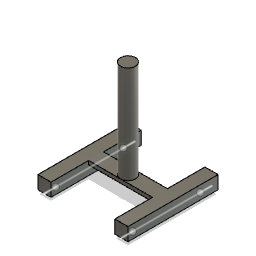
Pedestal (Autodesk Fusion 360 design; units mm, degrees)
Autodesk Fusion 360 part; units mm, degrees
sketch "Sketch1" plane through (0, 0, 0) normal (0, 1, 0) x (1, 0, 0)
  line L0 (609.6, 0) -> (609.6, 609.6)
  line L1 (0, 609.6) -> (0, 0)
  line L2 (0, 0) -> (88.9, 0)
  line L3 (88.9, 609.6) -> (0, 609.6)
  line L4 (0, 609.6) -> (0, 0)
  line L5 (609.6, 609.6) -> (520.7, 609.6)
  line L6 (520.7, -460.804) -> (609.6, -460.804)
  line L7 (609.6, -460.804) -> (609.6, 609.6)
  line L8 (609.6, 304.8) -> (609.6, 355.6)
  line L9 (520.7, 355.6) -> (88.9, 355.6)
  line L10 (0, 355.6) -> (0, 304.8)
  line L11 (609.6, 304.8) -> (609.6, 254)
  line L12 (520.7, 254) -> (88.9, 254)
  line L13 (0, 254) -> (0, 304.8)
  line L14 (88.9, 0) -> (88.9, 254)
  line L15 (88.9, 355.6) -> (88.9, 609.6)
  line L16 (520.7, 609.6) -> (520.7, 355.6)
  line L17 (520.7, 254) -> (520.7, 0)
  line L18 (0, 0) -> (88.9, 0)
  line L19 (520.7, 0) -> (609.6, 0)
  line L20 (609.6, 609.6) -> (520.7, 609.6)
  line L21 (88.9, 609.6) -> (0, 609.6)
  dimension "d1" = 609.6
  dimension "d2" = 609.6
  dimension "d3" = 88.9
  dimension "d4" = 88.9
  dimension "d5" = 50.8
  dimension "d6" = 50.8
  constraint horizontal L18
  constraint vertical L0
  constraint horizontal L20
  constraint vertical L1
  constraint coincident L1.end L2.start
  constraint horizontal L2
  constraint vertical L14
  constraint horizontal L3
  constraint vertical L4
  constraint horizontal L5
  constraint vertical L16
  constraint horizontal L6
  constraint vertical L7
  constraint midpoint L1 L10.end
  constraint vertical L8
  constraint horizontal L9
  constraint vertical L10
  constraint vertical L11
  constraint horizontal L12
  constraint vertical L13
  constraint collinear L14 L15
  constraint coincident L12.start L16
  constraint coincident L17.end L18
  constraint collinear L16 L17
  constraint collinear L18 L19
  constraint collinear L20 L21
  measures "d1" distance of L1.end L0.start
  measures "d2" distance of L1.end L1.start
  measures "d3" distance of L1.end L2.end
  measures "d4" distance of L0.end L5.end
  measures "d5" distance of L10.end L10.start
  measures "d6" distance of L10.end L13.start
extrude "Extrude1" add sketch "Sketch1" along normal blind 25.4
sketch "Sketch2" plane through (0, 0, 0) normal (0, -1, 0) x (1, 0, 0)
  line L0 (609.6, -609.6) -> (609.6, 0)
  line L1 (609.6, 0) -> (520.7, 0)
  line L2 (520.7, 0) -> (520.7, -254)
  line L3 (520.7, -254) -> (88.9, -254)
  line L4 (88.9, -254) -> (88.9, 0)
  line L5 (88.9, 0) -> (0, 0)
  line L6 (0, 0) -> (0, -609.6)
  line L7 (0, -609.6) -> (88.9, -609.6)
  line L8 (88.9, -609.6) -> (88.9, -355.6)
  line L9 (88.9, -355.6) -> (520.7, -355.6)
  line L10 (520.7, -355.6) -> (520.7, -609.6)
  line L11 (520.7, -609.6) -> (609.6, -609.6)
  line L12 (0, 0) -> (88.9, 0)
  line L13 (88.9, 0) -> (88.9, -609.6)
  line L14 (88.9, -609.6) -> (0, -609.6)
  line L15 (0, -609.6) -> (0, 0)
  line L16 (520.7, 0) -> (609.6, 0)
  line L17 (609.6, 0) -> (609.6, -609.6)
  line L18 (609.6, -609.6) -> (520.7, -609.6)
  line L19 (520.7, -609.6) -> (520.7, 0)
  constraint horizontal L12
  constraint vertical L13
  constraint horizontal L14
  constraint vertical L15
  constraint coincident L7.end L8.start
  constraint coincident L5.end L6.start
  constraint horizontal L16
  constraint vertical L17
  constraint horizontal L18
  constraint vertical L19
  constraint coincident L0.start L11.end
  constraint coincident L1.end L2.start
extrude "Extrude2" add sketch "Sketch2" along normal blind 63.5 contours L0 L1 L2 L10 L11 L16 L17 L18 L19 | L4 L5 L6 L7 L8 L12 L13 L14 L15
sketch "Sketch3" plane through (0, 25.4, 0) normal (0, 1, 0) x (-1, 0, 0)
  line L0 (-609.6, 0) -> (-609.6, -609.6)
  line L1 (-609.6, -609.6) -> (-520.7, -609.6)
  line L2 (-520.7, -609.6) -> (-520.7, -355.6)
  line L3 (-520.7, -355.6) -> (-88.9, -355.6)
  line L4 (-88.9, -355.6) -> (-88.9, -609.6)
  line L5 (-88.9, -609.6) -> (0, -609.6)
  line L6 (0, -609.6) -> (0, 0)
  line L7 (0, 0) -> (-88.9, 0)
  line L8 (-88.9, 0) -> (-88.9, -254)
  line L9 (-88.9, -254) -> (-520.7, -254)
  line L10 (-520.7, -254) -> (-520.7, 0)
  line L11 (-520.7, 0) -> (-609.6, 0)
  circle A0 centre (-304.8, -304.8) radius 50.8
  constraint tangent L3 A0
extrude "Extrude3" add sketch "Sketch3" along normal blind 762 contours A0
extrude "Extrude4" cut 1 faces at (289.3545, 787.4, -299.9767) along direction (0, -1, 0) blind 101.6
sketch "Sketch4" plane through (0, -63.5, 0) normal (0, -1, 0) x (1, 0, 0)
  line L0 (0, -609.6) -> (88.9, -609.6)
  line L1 (88.9, -609.6) -> (88.9, 0)
  line L2 (88.9, 0) -> (0, 0)
  line L3 (0, 0) -> (0, -609.6)
  line L4 (44.45, 0) -> (44.45, -609.6)
  line L5 (44.45, 0) -> (44.45, -11.9009)
  line L6 (44.45, 0) -> (44.45, -76.2)
  line L7 (44.45, -609.6) -> (44.45, -533.4)
  dimension "d15" = 76.2
  dimension "d16" = 76.2
  constraint midpoint L2 L4.start
  constraint midpoint L0 L4.end
  constraint coincident L4 L5.end
  constraint perpendicular L2 L5
  constraint perpendicular L2 L6
  constraint perpendicular L0 L7
  measures "d15" distance of L4.start L6.end
  measures "d16" distance of L4.end L7.end
sphere "SpherePrimitive1" add diameter 50.8 placed x (1, 0, 0) y (0, 0, 1) z (0, -1, 0) at (44.23, -63.5, -74.8157)
sphere "SpherePrimitive2" add diameter 50.8 placed x (1, 0, 0) y (0, 0, 1) z (0, -1, 0) at (44.8206, -63.5, -533.484)
sketch "Sketch7" plane through (0, -63.5, 0) normal (0, -1, 0) x (1, 0, 0)
  line L0 (520.7, -609.6) -> (609.6, -609.6)
  line L1 (609.6, -609.6) -> (609.6, 0)
  line L2 (609.6, 0) -> (520.7, 0)
  line L3 (520.7, 0) -> (520.7, -609.6)
  line L4 (565.15, 0) -> (565.15, -609.6)
  line L5 (565.15, 0) -> (565.15, -76.2)
  line L6 (565.15, -609.6) -> (565.15, -533.4)
  dimension "d19" = 76.2
  dimension "d20" = 76.2
  constraint midpoint L2 L4.start
  constraint midpoint L0 L4.end
  constraint perpendicular L2 L5
  constraint perpendicular L0 L6
  measures "d19" distance of L4.start L5.end
  measures "d20" distance of L4.end L6.end
sphere "SpherePrimitive3" add diameter 50.8 placed x (1, 0, 0) y (0, 0, 1) z (0, -1, 0) at (565.3152, -63.5, -75.9261)
sphere "SpherePrimitive4" add diameter 50.8 placed x (1, 0, 0) y (0, 0, 1) z (0, -1, 0) at (565.1233, -63.5, -532.8086)
